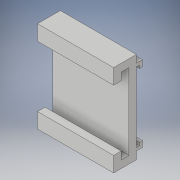
# Autodesk Inventor part: Substrategrip0degreesThick
Saved by Autodesk Inventor 2019 (Build 230136000, 136)
## iProperties
Created: 2018-09-07
Part Number: Substrategrip0degreesThick
Material: Generic
Document SubType Name: Modeling
Designer: s152529
Density: 1 g/cm^3
Appearance: Default
Author: s152529
Autodesk Inventor part; units mm, degrees
ref_plane "YZ Plane" through (0, 0, 0) normal (1, 0, 0) x (0, 1, 0)
ref_plane "XZ Plane" through (0, 0, 0) normal (0, 1, 0) x (-1, 0, 0)
ref_plane "XY Plane" through (0, 0, 0) normal (0, 0, 1) x (1, 0, 0)
sketch "Sketch1" plane through (0, 0, 0) normal (0, 0, 1) x (1, 0, 0)
  line L0 (-25, 30) -> (25, 30)
  line L1 (25, 30) -> (25, -30)
  line L2 (25, -30) -> (-25, -30)
  line L3 (-25, -30) -> (-25, 30)
  point P0 (0, 0)
  dimension "d0" = 50
  dimension "d1" = 60
  dimension "d2" = 30
  dimension "d3" = 25
  constraints: 8 end point, 2 parallel, 1 horizontal, 1 perpendicular
  measures "d0" distance of L1.end L2.end
  measures "d1" distance between parallel lines of L2 L0
  measures "d2" distance from line of L0 point (0, 0)
  measures "d3" distance from line of point (0, 0) L3
extrude "Extrusion1" add sketch "Sketch1" along normal blind 5
sketch "Sketch2" plane through (0, 0, 5) normal (0, 0, 1) x (1, 0, 0)
  line L0 (-25, 30) -> (-25, -30) projected
  line L1 (-25, 25) -> (25, 25)
  line L2 (25, -30) -> (25, 30) projected
  line L3 (25, 30) -> (-25, 30) projected
  point P0 (0, 0)
  dimension "d6" = 5
  constraints: 2 end point, 2 point on line, 1 horizontal
  measures "d6" distance between parallel lines of L3 L1
extrude "Extrusion2" add sketch "Sketch2" along normal blind 10
sketch "Sketch3" plane through (0, 0, 5) normal (0, 0, 1) x (1, 0, 0)
  line L0 (-25, -30) -> (-25, 30) projected
  line L1 (-25, -25) -> (25, -25)
  line L2 (25, 30) -> (25, -30) projected
  line L3 (-25, -30) -> (25, -30) projected
  point P0 (0, 0)
  dimension "d9" = 5
  constraints: 2 end point, 2 point on line, 1 horizontal
  measures "d9" distance between parallel lines of L3 L1
extrude "Extrusion3" add sketch "Sketch3" along normal blind 10
sketch "Sketch4" plane through (-25, -25, 5) normal (0, 1, 0) x (1, 0, 0)
  line L0 (0, 5) -> (0, -10) projected
  line L1 (0, -5) -> (50, -5)
  line L2 (50, 5) -> (50, -10) projected
  line L3 (0, -10) -> (50, -10) projected
  point P0 (25, 5)
  dimension "d12" = 5
  constraints: 2 end point, 2 point on line, 1 horizontal
  measures "d12" distance between parallel lines of L3 L1
extrude "Extrusion4" add sketch "Sketch4" along normal blind 5
sketch "Sketch5" plane through (-25, 25, 5) normal (0, -1, 0) x (1, 0, 0)
  line L0 (0, -5) -> (0, 10) projected
  line L1 (0, 5) -> (50, 5)
  line L2 (50, -5) -> (50, 10) projected
  line L3 (50, 10) -> (0, 10) projected
  point P0 (25, -5)
  dimension "d15" = 5
  constraints: 2 end point, 2 point on line, 1 horizontal
  measures "d15" distance between parallel lines of L3 L1
extrude "Extrusion5" add sketch "Sketch5" along normal blind 5
sketch "Sketch6" plane through (0, 0, 0) normal (0, 0, -1) x (-1, 0, 0)
  line L0 (-25, 30) -> (-25, -30) projected
  line L1 (25, -30) -> (25, 30) projected
  line L2 (-25, 25) -> (25, 25)
  line L3 (25, 25) -> (25, 23)
  line L4 (25, 23) -> (-25, 23)
  line L5 (-25, 23) -> (-25, 25)
  line L6 (25, 30) -> (-25, 30) projected
  point P0 (0, 0)
  dimension "d18" = 2
  dimension "d19" = 5
  constraints: 8 end point, 2 parallel, 2 point on line, 1 horizontal, 1 perpendicular
  measures "d18" distance between parallel lines of L4 L2
  measures "d19" distance between parallel lines of L6 L2
extrude "Extrusion6" add sketch "Sketch6" along normal blind 4 contours L2 L1 L4 L0
sketch "Sketch7" plane through (0, 0, 0) normal (0, 0, -1) x (-1, 0, 0)
  line L0 (-25, 23) -> (-25, -30) projected
  line L1 (25, -30) -> (25, 23) projected
  line L2 (-25, -25) -> (25, -25)
  line L3 (25, -25) -> (25, -23)
  line L4 (25, -23) -> (-25, -23)
  line L5 (-25, -23) -> (-25, -25)
  line L6 (-25, -30) -> (25, -30) projected
  point P0 (0, 0)
  dimension "d22" = 2
  dimension "d23" = 5
  constraints: 8 end point, 2 parallel, 2 point on line, 1 horizontal, 1 perpendicular
  measures "d22" distance between parallel lines of L2 L4
  measures "d23" distance between parallel lines of L6 L2
extrude "Extrusion7" add sketch "Sketch7" along normal blind 4 contours L4 L1 L2 L0
sketch "Sketch8" plane through (-25, 23, 0) normal (0, -1, 0) x (1, 0, 0)
  point P0 (25, 0)
sketch "Sketch9" plane through (-25, 23, 0) normal (0, -1, 0) x (1, 0, 0)
  line L0 (50, 0) -> (50, -4) projected
  line L1 (0, 0) -> (0, -4) projected
  line L2 (50, -4) -> (0, -4)
  line L3 (0, -4) -> (0, -2)
  line L4 (0, -2) -> (50, -2)
  line L5 (50, -2) -> (50, -4)
  point P0 (25, 0)
  constraints: 8 end point, 2 parallel, 1 horizontal, 1 midpoint, 1 perpendicular
extrude "Extrusion8" add sketch "Sketch9" along normal blind 2
sketch "Sketch10" plane through (-25, -23, 0) normal (0, 1, 0) x (1, 0, 0)
  line L0 (0, 0) -> (0, 4) projected
  line L1 (50, 0) -> (50, 4) projected
  line L2 (0, 4) -> (50, 4)
  line L3 (50, 4) -> (50, 2)
  line L4 (50, 2) -> (0, 2)
  line L5 (0, 2) -> (0, 4)
  point P0 (25, 0)
  constraints: 8 end point, 2 parallel, 1 horizontal, 1 midpoint, 1 perpendicular
extrude "Extrusion9" add sketch "Sketch10" along normal blind 2
body "Solid1"
